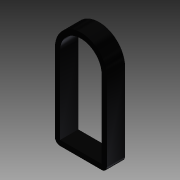
# Autodesk Inventor part: ZIP TIE GANTRY ROD
Saved by Autodesk Inventor 2013 (Build 170138000, 138)
## iProperties
Created: 2014-06-21
Part Number: ZIP TIE GANTRY ROD
Material: Generic
Document SubType Name: Modeling
Designer: employee
Density: 1 g/cm^3
Author: employee
Autodesk Inventor part; units mm, degrees
ref_plane "YZ Plane" through (0, 0, 0) normal (1, 0, 0) x (0, 1, 0)
ref_plane "XZ Plane" through (0, 0, 0) normal (0, 1, 0) x (-1, 0, 0)
ref_plane "XY Plane" through (0, 0, 0) normal (0, 0, 1) x (1, 0, 0)
sketch "Sketch1" plane through (0, 0, 0) normal (0, 0, 1) x (1, 0, 0)
  line L0 (1.5, -5.715) -> (0, -5.715) construction
  line L1 (1.5, 0) -> (1.5, -5.715) construction
  line L2 (0, 0) -> (1.5, 0) construction
  line L3 (0, 0) -> (0, -5.715) construction
  line L4 (1.5, 0) -> (0, 0) construction
  line L5 (1.5, 5.715) -> (1.5, 0) construction
  line L6 (0, 5.715) -> (1.5, 5.715) construction
  line L7 (0, 5.715) -> (0, 0) construction
  line L8 (-8, 0) -> (-9.5, 0) construction
  line L9 (-8, 5.715) -> (-8, 0) construction
  line L10 (-9.5, 5.715) -> (-8, 5.715) construction
  line L11 (-9.5, 5.715) -> (-9.5, 0) construction
  line L12 (-8, -5.715) -> (-9.5, -5.715) construction
  line L13 (-8, 0) -> (-8, -5.715) construction
  line L14 (-9.5, 0) -> (-8, 0) construction
  line L15 (-9.5, 0) -> (-9.5, -5.715) construction
  circle A0 centre (-4, 9.1791) radius 4 construction
  line L16 (-8, -5.715) -> (-8, 9.1791)
  line L17 (0, -5.715) -> (0, 9.1791)
  line L18 (0, -5.715) -> (-8, -5.715)
  arc A1 (0, 9.1791) -> (-8, 9.1791) centre (-4, 9.1791) ccw
  line L19 (-9, 9.1791) -> (-9, -6.715)
  line L20 (-9, -6.715) -> (1, -6.715)
  line L21 (1, -6.715) -> (1, 9.1791)
  arc A2 (1, 9.1791) -> (-9, 9.1791) centre (-4, 9.1791) ccw
  dimension "d0" = 1
  constraints: 12 end point, 6 point on circle, 4 tangent, 2 centre point, 2 perpendicular, 3 other
  measures "d0" distance between parallel lines of L20 L18
extrude "Extrusion1" add sketch "Sketch1" along normal blind 3.5
fillet "Fillet1" radius 1 2 edges at (-9, -6.715, 1.75) (1, -6.715, 1.75)
body "Solid1"
